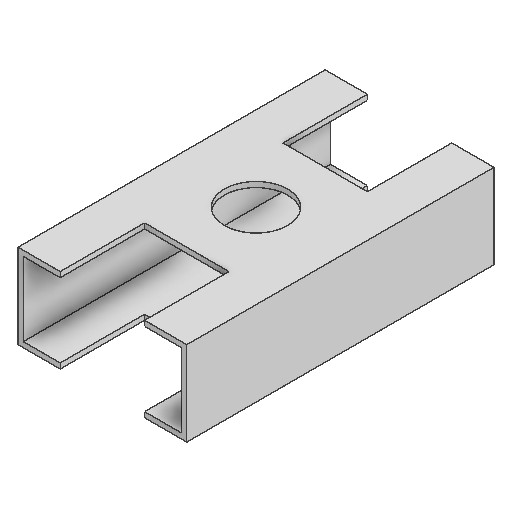
# Autodesk Inventor part: Diff Top Bar
Saved by Autodesk Inventor 2025.2 (Build 292293000, 293)
## iProperties
Created: 2025-02-20
Part Number: Diff Top Bar
Material: Generic
Document SubType Name: Modeling
Designer: Jakeg
Density: 1 g/cm^3
Appearance: Default
Author: Jakeg
Autodesk Inventor part; units mm, degrees
ref_plane "YZ Plane" through (0, 0, 0) normal (1, 0, 0) x (0, 1, 0)
ref_plane "XZ Plane" through (0, 0, 0) normal (0, 1, 0) x (-1, 0, 0)
ref_plane "XY Plane" through (0, 0, 0) normal (0, 0, 1) x (1, 0, 0)
sketch "Sketch1" plane through (0, 0, 0) normal (0, 0, 1) x (1, 0, 0)
  line L0 (-15.6216, 9.2219) -> (35.1784, 9.2219)
  line L1 (35.1784, 9.2219) -> (35.1784, -16.1781)
  line L2 (35.1784, -16.1781) -> (-15.6216, -16.1781)
  line L3 (-15.6216, -16.1781) -> (-15.6216, 9.2219)
  line L4 (-14.0341, 7.6344) -> (33.5909, 7.6344)
  line L5 (33.5909, 7.6344) -> (33.5909, -14.5906)
  line L6 (33.5909, -14.5906) -> (-14.0341, -14.5906)
  line L7 (-14.0341, -14.5906) -> (-14.0341, 7.6344)
  point P0 (0, 0)
  dimension "d0" = 50.8
  dimension "d1" = 25.4
  dimension "d2" = 1.5875
  dimension "d3" = 1.5875
  dimension "d4" = 1.5875
  dimension "d5" = 1.5875
  constraints: 16 end point, 4 parallel, 2 horizontal, 2 perpendicular
  measures "d0" distance of L0.start L0.end
  measures "d1" distance of L0.end L1.end
  measures "d2" distance between parallel lines of L3 L7
  measures "d3" distance between parallel lines of L1 L5
  measures "d4" distance between parallel lines of L2 L6
  measures "d5" distance between parallel lines of L0 L4
extrude "Extrusion1" add sketch "Sketch1" along normal blind 92.456
sketch "Sketch2" plane through (-15.6216, 9.2219, 0) normal (0, 1, 0) x (1, 0, 0)
  circle A0 centre (25.4, -46.228) radius 9.4996
  line L0 (0, 0) -> (0, -92.456) projected
  line L1 (50.8, 0) -> (0, 0) projected
  line L2 (12.7, 0) -> (38.1, 0)
  line L3 (38.1, 0) -> (38.1, -25.4)
  line L4 (38.1, -25.4) -> (12.7, -25.4)
  line L5 (12.7, -25.4) -> (12.7, 0)
  line L6 (1.5875, -92.456) -> (49.2125, -92.456) projected
  line L7 (12.7, -92.456) -> (38.1, -92.456)
  line L8 (38.1, -92.456) -> (38.1, -67.056)
  line L9 (38.1, -67.056) -> (12.7, -67.056)
  line L10 (12.7, -67.056) -> (12.7, -92.456)
  point P0 (15.6216, 0)
  point P1 (25.4, -25.4)
  dimension "d8" = 18.9992
  dimension "d9" = 25.4
  dimension "d10" = 46.228
  dimension "d13" = 25.4
  dimension "d14" = 25.4
  dimension "d15" = 25.4
  dimension "d16" = 25.4
  constraints: 16 end point, 4 parallel, 2 horizontal, 2 perpendicular, 2 point on line, 1 centre point, 1 midpoint
  measures "d8" diameter of A0
  measures "d9" distance from line of L0 A0.centre
  measures "d10" distance from line of L1 A0.centre
  measures "d13" distance of L3.end L4.end
  measures "d14" distance of L2.end L3.end
  measures "d15" distance from line of L0 point (25.4, -25.4)
  measures "d16" distance of L8.end L7.end
extrude "Extrusion2" cut sketch "Sketch2" against normal blind 116.84
equation "\"d3\" = d2"
equation "\"d4\" = d2"
equation "\"d5\" = d2"
body "Solid1"
